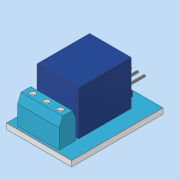
# Autodesk Inventor part: RelayModule
Saved by Autodesk Inventor 2017 (Build 210142000, 142)
## iProperties
Created: 2018-02-24
Part Number: RelayModule
Material: ABS Plastic
Document SubType Name: Modeling
Designer: Derek Wider
Density: 1.06 g/cm^3
Appearance: Smooth - White
Author: Derek Wider
Autodesk Inventor part; units mm, degrees
ref_plane "YZ Plane" through (0, 0, 0) normal (1, 0, 0) x (0, 1, 0)
ref_plane "XZ Plane" through (0, 0, 0) normal (0, 1, 0) x (-1, 0, 0)
ref_plane "XY Plane" through (0, 0, 0) normal (0, 0, 1) x (1, 0, 0)
sketch "Sketch1" plane through (0, 0, 0) normal (0, 1, 0) x (-1, 0, 0)
  line L0 (0, 0) -> (23.5, 0)
  line L1 (23.5, 0) -> (23.5, -33)
  line L2 (23.5, -33) -> (0, -33)
  line L3 (0, -33) -> (0, 0)
  dimension "d0" = 33
  dimension "d1" = 23.5
  constraints: 8 end point, 2 parallel, 1 horizontal, 1 perpendicular
  measures "d0" distance of L2.end L0.start
  measures "d1" distance of L1.end L2.end
extrude "Extrusion1" add sketch "Sketch1" along normal blind 2
sketch "Sketch2" plane through (0, 2, 0) normal (0, 1, 0) x (1, 0, 0)
  line L0 (-20.5, 8) -> (-5.5, 8)
  line L1 (-5.5, 8) -> (-5.5, 27)
  line L2 (-5.5, 27) -> (-20.5, 27)
  line L3 (-20.5, 27) -> (-20.5, 8)
  line L4 (-23.5, 0) -> (0, 0) construction
  line L5 (0, 0) -> (0, 33) construction
  line L6 (0, 33) -> (-23.5, 33) construction
  line L7 (-23.5, 33) -> (-23.5, 0) construction
  line L8 (-20.5, 8) -> (-23.5, 8) construction
  line L9 (-23.5, 33) -> (-23.5, 0) construction
  line L10 (-5.5, 8) -> (0, 8) construction
  dimension "d4" = 15
  dimension "d5" = 19
  dimension "d6" = 8
  dimension "d36" = 5.5
  constraints: 12 end point, 3 point on line, 2 parallel, 2 perpendicular, 1 horizontal
  measures "d4" distance of L0.start L0.end
  measures "d5" distance of L2.end L0.start
  measures "d6" distance between parallel lines of L4 L0
  measures "d36" distance of L0.end L10.end
extrude "Extrusion2" add sketch "Sketch2" along normal blind 16
sketch "Sketch3" plane through (0, 2, 0) normal (0, 1, 0) x (1, 0, 0)
  line L0 (-9, 31) -> (-16.5, 31)
  line L1 (-16.5, 31) -> (-16.5, 28.5)
  line L2 (-16.5, 28.5) -> (-9, 28.5)
  line L3 (-9, 28.5) -> (-9, 31)
  line L4 (-16.5, 28.5) -> (-23.5, 28.5) construction
  line L5 (-23.5, 33) -> (-23.5, 0) construction
  line L6 (-9, 28.5) -> (-2, 28.5) construction
  line L7 (0, 33) -> (-23.5, 33) construction
  line L8 (-10.625, 29.5) -> (-10.125, 29.5)
  line L9 (-10.125, 29.5) -> (-10.125, 30)
  line L10 (-10.125, 30) -> (-10.625, 30)
  line L11 (-10.625, 30) -> (-10.625, 29.5)
  line L12 (-13.125, 29.5) -> (-12.625, 29.5)
  line L13 (-12.625, 29.5) -> (-12.625, 30)
  line L14 (-12.625, 30) -> (-13.125, 30)
  line L15 (-13.125, 30) -> (-13.125, 29.5)
  line L16 (-15.625, 29.5) -> (-15.125, 29.5)
  line L17 (-15.125, 29.5) -> (-15.125, 30)
  line L18 (-15.125, 30) -> (-15.625, 30)
  line L19 (-15.625, 30) -> (-15.625, 29.5)
  line L20 (-10.125, 29.5) -> (-10.125, 28.5) construction
  line L21 (-10.125, 30) -> (-10.125, 31) construction
  point P0 (0, 0)
  dimension "d9" = 2
  dimension "d10" = 2.5
  dimension "d11" = 7.5
  dimension "d12" = 0.5
  dimension "d13" = 0.5
  dimension "d16" = 2.5
  dimension "d21" = 1.125
  dimension "d39" = 7
  constraints: 40 end point, 5 horizontal, 4 parallel, 4 point on line, 2 collinear, 2 perpendicular, 1 vertical, 16 other
  measures "d9" distance between parallel lines of L7 L0
  measures "d10" distance of L2.end L0.start
  measures "d11" distance of L1.end L2.end
  measures "d12" distance of L10.end L9.end
  measures "d13" distance of L9.end L8.end
  measures "d16" distance of L8.start L12.start
  measures "d21" distance between parallel lines of L3 L9
  measures "d39" distance between parallel lines of L5 L1
extrude "Extrusion3" add sketch "Sketch3" along normal blind 1.75
sketch "Sketch4" plane through (-5.5, 2, -8) normal (1, 0, 0) x (0, 0, -1)
  line L0 (-8, 0) -> (25, 0) construction
  line L1 (0, 0) -> (0, 16) construction
  line L2 (-1, 0) -> (-1, 7)
  line L3 (-1, 7) -> (-2.25, 10)
  line L4 (-2.25, 10) -> (-5.75, 10)
  line L5 (-5.75, 10) -> (-7, 7)
  line L6 (-7, 7) -> (-7, 0)
  line L7 (25, 0) -> (-8, 0) projected
  line L8 (-7, 0) -> (-1, 0)
  line L9 (-8, -2) -> (-8, 0) projected
  dimension "d26" = 6
  dimension "d27" = 10
  dimension "d28" = 3
  dimension "d37" = 1
  dimension "d38" = 3.5
  constraints: 12 end point, 3 perpendicular, 2 equal length, 2 point on line, 1 horizontal
  measures "d26" distance between parallel lines of L6 L2
  measures "d27" distance between parallel lines of L0 L4
  measures "d28" distance from line of L5.end L4
  measures "d37" distance between parallel lines of L9 L6
  measures "d38" distance of L3.end L4.end
extrude "Extrusion5" add sketch "Sketch4" against normal up to surface (15 mm away)
sketch "Sketch5" plane through (-5.5, 12, -2.25) normal (0, 1, 0) x (1, 0, 0)
  line L0 (0, 0) -> (-15, 0) construction
  circle A0 centre (-2.5, 1.6688) radius 1
  circle A1 centre (-7.5, 1.6688) radius 1
  circle A2 centre (-12.5, 1.6688) radius 1
  line L1 (-12.5, 1.6688) -> (-15, 1.6688) construction
  line L2 (-2.5, 1.6688) -> (0, 1.6688) construction
  line L3 (-15, 3.5) -> (-15, 0) construction
  line L4 (0, 3.5) -> (0, 0) construction
  point P0 (5.5, -2.25)
  dimension "d31" = 2
  dimension "d32" = 5
  dimension "d33" = 5
  constraints: 4 end point, 3 centre point, 2 equal radius, 2 horizontal, 2 point on line, 1 collinear
  measures "d31" diameter of A0
  measures "d32" distance of L1.start A1.centre
  measures "d33" distance of A1.centre L2.start
extrude "Extrusion6" cut sketch "Sketch5" against normal blind 1
sketch "Sketch6" plane through (-9, 2, -28.5) normal (1, 0, 0) x (0, 0, -1)
  line L0 (-28.5, 0) -> (4.5, 0) construction
  line L1 (2.5, 0) -> (2.5, 1.75) construction
  line L2 (0, 0) -> (0, 1.75) construction
  line L3 (1, 0) -> (1.5, 0) projected
  line L4 (1.25, 0) -> (1.25, 2)
  arc A0 (2.25, 3) -> (1.25, 2) centre (2.25, 2) ccw
  line L5 (2.25, 3) -> (8.25, 3)
  point P0 (-28.5, -2)
  dimension "d40" = 2
  dimension "d41" = 6
  dimension "d42" = 1
  constraints: 4 end point, 2 point on circle, 2 tangent, 1 centre point, 1 horizontal, 1 midpoint, 1 perpendicular
  measures "d40" distance of L4.start L4.end
  measures "d41" distance of L5.start L5.end
  measures "d42" radius of A0
sweep "Sweep1" add profiles "Sketch3" path "Sketch6" path curves L4 A0 L5 contours L11 L10 L9 L8 | L15 L14 L13 L12 | L19 L18 L17 L16
body "Solid1"
